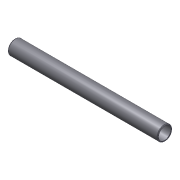
# Autodesk Inventor part: 04R-8.25550
Saved by Autodesk Inventor 2012 (Build 160160000, 160)
## iProperties
Category: PARTsolutions
Created: 2013-01-19
Part Number: 04R-8.25550
Catalog Web Link: www.cadenas.de
Description: Tube - Original Line - Standard Air Cylinders
Document SubType Name: Modeling
Designer: PARTsolutions
Material: Stainless Steel
Density: 8.08 g/cm^3
Mass: 62.6216 g
Surface Area: 265.131 cm^2
Volume: 7.75019 cm^3
NB: 04R-8.25550
NN: Tube
NT: Original Line - Standard Air Cylinders
NBSYN: $PN.
LINA: 04R-8.25550
PN: 04R-8.25550
BORE: 0.75000000
BOREPN: 04
MNTALG: '' , 'Front Nose' , 'BF' , 'Front Block' , 'BFT' , 'Front Trunnion' , 'A' , 'Adjustable Stroke'
ACTING: R
ACTINGALG: '' , 'Single Acting' , 'R' , 'Reverse/Double Acting'
NRALG: '' , 'N/A'
L: 8.2555
OD: 0.8075
ODN: 0.8050
ODP: 0.8625
ODB: 0.8325
ID: 0.7615
DV: 0.00000000
LV: 0.00000000
LV1: 0.00000000
G: 0.0300
FOURHOLES: 0
AA: 0.3750
BB: 0.0940
SRALG: 'C' , 'Carbon Steel Rod' , 'SR' , '303 Stainless Steel Rod' , '' , '303 Stainless Steel Rod'
KT: DUMMY
SUPPLIER: Bimba
ARTICLENO: 04R-8.25550
BOMINFO: 04R-8.25550
CREATOR: CADENAS GmbH
PSOL_IDENT_0: {\\10.0.0.242\data_v9\23d-libs\bimba\bimba\bimba_imperial\bimba_full_line\original_line_cylinders\st
PSOL_IDENT_1: andard_air_cylinders\tube.prj},190 {VTYP=3D},{NB=04R-8.25550},{LINA=04R-8.25550},{NN=Tube},{DATE=20.
PSOL_IDENT_2: 08.2011 07:16:50},{GEOMDATE=18.02.2011 00:00:00},{VERSION=},{LINEID=40},{LINESUBID=-1},{WBVAR=MNT,AC
PSOL_IDENT_3: TING,NR,L,FOURHOLES,SR}  {NB=04R-8.25550},{LINA=04R-8.25550},{KT=DUMMY},{PN=04R-8.25550},{BORE=0.750
PSOL_IDENT_4: 00000},{BOREPN=04},{MNT=},{MNTALG='' , 'Front Nose' , 'BF' , 'Front Block' , 'BFT' , 'Front Trunnion
PSOL_IDENT_5: ' , 'A' , 'Adjustable Stroke'},{ACTING=R},{ACTINGALG= '' , 'Single Acting' , 'R' , 'Reverse/Double A
PSOL_IDENT_6: cting' },{NR=},{NRALG= '' , 'N/A' },{L=8.2555},{OD=0.8075},{ODN=0.8050},{ODP=0.8625},{ODB=0.8325},{I
PSOL_IDENT_7: D=0.7615},{DV=0.00000000},{LV=0.00000000},{LV1=0.00000000},{G=0.0300},{FOURHOLES=0},{AA=0.3750},{BB=
PSOL_IDENT_8: 0.0940},{SR=},{SRALG= 'C' , 'Carbon Steel Rod' , 'SR' , '303 Stainless Steel Rod' , '' , '303 Stainl
PSOL_IDENT_9: ess Steel Rod'}
Title: 04R-8.25550
Author: Cadenas PARTsolutions
Comments: Original Line - Standard Air Cylinders
Autodesk Inventor part; units mm, degrees
sketch "Sketch_1" plane through (0, 0, 0) normal (0, 0, 1) x (1, 0, 0)
  line L0 (209.6897, 0) -> (0, 0)
  arc A0 (-0.6395, 9.3472) -> (-0.6395, 9.1676) centre (-0.5497, 9.2574) ccw
  line L1 (-0.6395, 9.1676) -> (-0.381, 8.9091)
  line L2 (-0.381, 8.9091) -> (0, 8.9091)
  line L3 (0, 8.9091) -> (0.762, 9.671)
  line L4 (0.762, 9.671) -> (208.9277, 9.671)
  line L5 (208.9277, 9.671) -> (209.6897, 8.9091)
  line L6 (209.6897, 8.9091) -> (210.0707, 8.9091)
  line L7 (210.0707, 8.9091) -> (210.3292, 9.1676)
  arc A1 (210.3292, 9.1676) -> (210.3292, 9.3472) centre (210.2394, 9.2574) ccw
  line L8 (210.3292, 9.3472) -> (209.6443, 10.0321)
  arc A2 (209.6443, 10.0321) -> (209.1055, 10.2553) centre (209.1055, 9.4933) ccw
  line L9 (209.1055, 10.2553) -> (0.5842, 10.2553)
  arc A3 (0.5842, 10.2553) -> (0.0454, 10.0321) centre (0.5842, 9.4933) ccw
  line L10 (0.0454, 10.0321) -> (-0.6395, 9.3472)
  constraints: 22 end point, 8 point on circle, 4 centre point
revolve "Revolution1" add sketch "Sketch_1" angle 360 about axis through (209.6897, 0, 0) along (1, 0, 0)
ref_plane "tube_front_XY" through (0, 0, 0) normal (1, 0, 0) x (0, 0, -1)
ref_plane "tube_front_YZ" through (0, 0, 0) normal (0, 0, -1) x (0, 1, 0)
ref_plane "tube_front_ZX" through (0, 0, 0) normal (0, 1, 0) x (1, 0, 0)
ref_plane "tube_rear_XY" through (209.6897, 0, 0) normal (1, 0, 0) x (0, 0, -1)
ref_plane "tube_rear_YZ" through (209.6897, 0, 0) normal (0, 0, -1) x (0, 1, 0)
ref_plane "tube_rear_ZX" through (209.6897, 0, 0) normal (0, 1, 0) x (1, 0, 0)
ref_plane "cp1_XY" through (104.8448, 10.2553, 0) normal (1, 0, 0) x (0, 0, -1)
ref_plane "cp1_YZ" through (104.8448, 10.2553, 0) normal (0, 0, -1) x (0, 1, 0)
ref_plane "cp1_ZX" through (104.8448, 10.2553, 0) normal (0, 1, 0) x (1, 0, 0)
ref_plane "cp2_XY" through (104.8448, 0, -10.2553) normal (1, 0, 0) x (0, 0, -1)
ref_plane "cp2_YZ" through (104.8448, 0, -10.2553) normal (0, 0, -1) x (0, 1, 0)
ref_plane "cp2_ZX" through (104.8448, 0, -10.2553) normal (0, 1, 0) x (1, 0, 0)
ref_plane "cp3_XY" through (104.8448, -10.2553, 0) normal (1, 0, 0) x (0, 0, -1)
ref_plane "cp3_YZ" through (104.8448, -10.2553, 0) normal (0, 0, -1) x (0, 1, 0)
ref_plane "cp3_ZX" through (104.8448, -10.2553, 0) normal (0, 1, 0) x (1, 0, 0)
ref_plane "cp4_XY" through (104.8448, 0, 10.2553) normal (1, 0, 0) x (0, 0, -1)
ref_plane "cp4_YZ" through (104.8448, 0, 10.2553) normal (0, 0, -1) x (0, 1, 0)
ref_plane "cp4_ZX" through (104.8448, 0, 10.2553) normal (0, 1, 0) x (1, 0, 0)
body "Solid1"
